11 slot compliant hex bit holder (Autodesk Fusion 360 design; units mm, degrees)
Autodesk Fusion 360 part; units mm, degrees
sketch "Sketch1" plane through (0, 0, 0) normal (0, 0, 1) x (1, 0, 0)
  line L0 (3.7239, 0) -> (1.862, 3.225)
  line L1 (1.862, 3.225) -> (-1.862, 3.225)
  line L2 (-1.862, 3.225) -> (-3.7239, 0)
  line L3 (-3.7239, 0) -> (-1.862, -3.225)
  line L4 (-1.862, -3.225) -> (1.862, -3.225)
  line L5 (1.862, -3.225) -> (3.7239, 0)
  line L6 (-4.8786, 0) -> (-2.4393, -4.225)
  line L7 (-2.4393, -4.225) -> (2.4393, -4.225)
  line L8 (2.4393, -4.225) -> (4.8786, 0)
  line L9 (4.8786, 0) -> (2.4393, 4.225)
  line L10 (2.4393, 4.225) -> (-2.4393, 4.225)
  line L11 (-2.4393, 4.225) -> (-4.8786, 0)
  line L12 (0.5, -3.225) -> (0.5, -3.075)
  line L13 (0, -3.225) -> (0, -3.5791) construction
  line L14 (-0.5, -3.225) -> (-0.5, -3.075)
  line L15 (0.5, -3.075) -> (-0.5, -3.075)
  arc A0 (0.5, -4.225) -> (-0.5, -4.225) centre (0, -4.225) ccw
  dimension "d1" = 6.45
  dimension "d2" = 1
  dimension "d3" = 1
  dimension "d4" = 6.3
  dimension "d5" = 0.5
  constraint horizontal L4
  constraint coincident L4 L12.start
  constraint perpendicular L4 L12
  constraint midpoint L4 L13.start
  constraint perpendicular L4 L13
  constraint symmetric L12.start L13 L14.start
  constraint symmetric L12.end L13 L14.end
  constraint perpendicular L14 L15
  constraint coincident L7 A0.end
  constraint coincident L7 A0.start
  constraint midpoint L7 A0.centre
  measures "d1" distance of L2 L5
  measures "d3" distance of L12.end L14.end
  measures "d4" distance of L1 L15
  measures "d5" radius of A0
extrude "Extrude1" add sketch "Sketch1" along normal blind 2 contours L0 L1 L2 L3 L4 L5 L12 L14 L15 | L4 L12 L14 L15 makes body 1
extrude "Extrude2" add sketch "Sketch1" along normal blind 12 contours L4 L12 L14 L15 | L6 L7 L8 L9 L10 L11 A0 bodies 1
sketch "Sketch2" plane through (0, -3.075, 0) normal (0, 1, 0) x (-1, 0, 0)
  line L0 (0.5, 2) -> (1.862, 2)
  line L1 (1.862, 2) -> (1.862, 12)
  line L2 (1.862, 12) -> (0.5, 12)
  line L3 (-1.862, 12) -> (-1.862, 2)
  line L4 (-1.181, 2) -> (-1.181, 2.3)
  line L5 (1.181, 2.3) -> (1.181, 2)
  line L6 (1.181, 2.3) -> (1.038, 2.3)
  line L7 (1.038, 2.3) -> (-1.181, 2.3)
  line L8 (-0.5, 2) -> (0.5, 2)
  line L9 (0.5, 12) -> (0.5, 2)
  line L10 (-1.862, 2) -> (-0.5, 2)
  line L11 (-0.5, 2) -> (-0.5, 12)
  line L12 (-0.5, 12) -> (-1.862, 12)
  line L13 (-0.5, 2) -> (0.5, 2)
  line L14 (0.5, 2) -> (0.5, 12)
  line L15 (0.5, 12) -> (-0.5, 12)
  line L16 (-0.5, 12) -> (-0.5, 2)
  dimension "d10" = 0.3
  constraint midpoint L0 L5.end
  constraint perpendicular L0 L5
  constraint perpendicular L5 L6
  constraint perpendicular L4 L7
  constraint coincident L0.start L8.end
  measures "d10" distance of L4.start L4.end
extrude "Extrude3" cut sketch "Sketch2" against normal through all contours L0 L5 L6 L7 L9 L14 | L7 L8 L9 L11 L13 L14 L16 | L4 L7 L10 L11 L16 bodies 1
chamfer "Chamfer2" distance 0.5 distance2 0.4 7 edges at (1.181, -3.225, 12) (-1.181, -3.225, 12) (-2.7929, -1.6125, 12) (-2.7929, 1.6125, 12) (0, 3.225, 12) (2.7929, 1.6125, 12) (2.7929, -1.6125, 12) measured on face at (-3.6806, 1.4083, 12) measured on face at (-3.6806, 1.4083, 12) measured on face at (-3.6806, 1.4083, 12) measured on face at (-3.6806, 1.4083, 12) measured on face at (-3.6806, 1.4083, 12) measured on face at (-3.6806, 1.4083, 12) measured on face at (-3.6806, 1.4083, 12) on bodies 1
chamfer "Chamfer1" distance 0.6 distance2 0.4 1 edges at (0, -3.075, 12) measured on face at (-0.0125, -3.2921, 12) on bodies 1
chamfer "Chamfer3" distance 0.15 distance2 0.15 1 edges at (0, -3.075, 2.3) measured on face at (0.1667, -3.075, 5.4) on bodies 1
pattern_linear "R-Pattern1" count 11 spacing 9.5 along (1, 0, 0) of bodies 1 makes body 2 at (9.5125, 1.5745, 0) makes body 3 at (19.0125, 1.5745, 0) makes body 4 at (28.5125, 1.5745, 0) makes body 5 at (38.0125, 1.5745, 0) makes body 6 at (47.5125, 1.5745, 0) makes body 7 at (57.0125, 1.5745, 0) makes body 8 at (66.5125, 1.5745, 0) makes body 9 at (76.0125, 1.5745, 0) makes body 10 at (85.5125, 1.5745, 0) makes body 11 at (95.0125, 1.5745, 0)
sketch "Sketch3" plane through (0, 0, 0) normal (0, 0, 1) x (1, 0, 0)
  line L0 (97.4393, 4.225) -> (-2.4393, 4.225)
  line L1 (97.4393, -4.225) -> (-2.4393, -4.225)
  line L2 (97.4393, -4.225) -> (97.4393, 4.225)
  line L3 (-2.4393, -4.225) -> (-2.4393, 4.225)
  line L4 (4.8786, 0) -> (2.4393, 4.225)
  line L5 (7.0607, 4.225) -> (4.6214, 0)
  line L6 (2.4393, -4.225) -> (4.8786, 0)
  line L7 (4.6214, 0) -> (7.0607, -4.225)
  line L8 (14.3786, 0) -> (11.9393, 4.225)
  line L9 (16.5607, 4.225) -> (14.1214, 0)
  line L10 (11.9393, -4.225) -> (14.3786, 0)
  line L11 (14.1214, 0) -> (16.5607, -4.225)
  line L12 (23.8786, 0) -> (21.4393, 4.225)
  line L13 (26.0607, 4.225) -> (23.6214, 0)
  line L14 (21.4393, -4.225) -> (23.8786, 0)
  line L15 (23.6214, 0) -> (26.0607, -4.225)
  line L16 (33.3786, 0) -> (30.9393, 4.225)
  line L17 (30.9393, -4.225) -> (33.3786, 0)
  line L18 (33.1214, 0) -> (35.5607, -4.225)
  line L19 (35.5607, 4.225) -> (33.1214, 0)
  line L20 (45.0607, 4.225) -> (42.6214, 0)
  line L21 (42.8786, 0) -> (40.4393, 4.225)
  line L22 (40.4393, -4.225) -> (42.8786, 0)
  line L23 (42.6214, 0) -> (45.0607, -4.225)
  line L24 (49.9393, -4.225) -> (52.3786, 0)
  line L25 (52.1214, 0) -> (54.5607, -4.225)
  line L26 (52.3786, 0) -> (49.9393, 4.225)
  line L27 (54.5607, 4.225) -> (52.1214, 0)
  line L28 (61.8786, 0) -> (59.4393, 4.225)
  line L29 (64.0607, 4.225) -> (61.6214, 0)
  line L30 (59.4393, -4.225) -> (61.8786, 0)
  line L31 (61.6214, 0) -> (64.0607, -4.225)
  line L32 (68.9393, -4.225) -> (71.3786, 0)
  line L33 (71.3786, 0) -> (68.9393, 4.225)
  line L34 (73.5607, 4.225) -> (71.1214, 0)
  line L35 (71.1214, 0) -> (73.5607, -4.225)
  line L36 (78.4393, -4.225) -> (80.8786, 0)
  line L37 (80.8786, 0) -> (78.4393, 4.225)
  line L38 (83.0607, 4.225) -> (80.6214, 0)
  line L39 (80.6214, 0) -> (83.0607, -4.225)
  line L40 (87.9393, -4.225) -> (90.3786, 0)
  line L41 (90.1214, 0) -> (92.5607, -4.225)
  line L42 (90.3786, 0) -> (87.9393, 4.225)
  line L43 (92.5607, 4.225) -> (90.1214, 0)
  point P0 (-2.4393, -4.225)
  point P1 (97.4393, -4.225)
  point P2 (97.4393, 4.225)
  point P3 (-2.4393, 4.225)
  constraint coincident P2 L0.start
  constraint coincident P3 L0.end
  constraint coincident P1 L1.start
  constraint coincident P0 L1.end
extrude "Extrude4" add sketch "Sketch3" along normal blind 2 bodies 1 2 3 4 5 6 7 8 9 10 11
extrude "Extrude5" add sketch "Sketch3" along normal blind 12 contours L0 L42 L43 | L1 L40 L41 | L0 L37 L38 | L1 L36 L39 | L0 L33 L34 | L1 L32 L35 | L0 L28 L29 | L1 L30 L31 | L0 L26 L27 | L1 L24 L25 | L0 L20 L21 | L1 L22 L23 | L0 L16 L19 | L1 L17 L18 | L0 L12 L13 | L1 L14 L15 | L0 L8 L9 | L1 L10 L11 | L0 L4 L5 | L1 L6 L7 bodies 1
